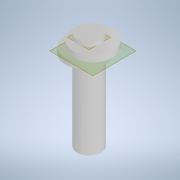
# Autodesk Inventor part: input_shaft
Saved by Autodesk Inventor 2022 (Build 260153000, 153)
## iProperties
Created: 2021-07-18
Part Number: input_shaft
Material: Generic
Document SubType Name: Modeling
Designer: Madhav
Density: 1 g/cm^3
Appearance: Default
Author: Madhav
Autodesk Inventor part; units mm, degrees
ref_plane "YZ Plane" through (0, 0, 0) normal (1, 0, 0) x (0, 1, 0)
ref_plane "XZ Plane" through (0, 0, 0) normal (0, 1, 0) x (-1, 0, 0)
ref_plane "XY Plane" through (0, 0, 0) normal (0, 0, 1) x (1, 0, 0)
sketch "Sketch1" plane through (0, 0, 0) normal (0, 1, 0) x (-1, 0, 0)
  point P0 (0, 0)
sketch "Sketch2" plane through (0, 0, 0) normal (0, 1, 0) x (-1, 0, 0)
  circle A0 centre (0, 0) radius 6
  dimension "d20" = 12
  constraints: 1 centre point, 1 coincident
  measures "d20" diameter of A0
extrude "Extrusion1" add sketch "Sketch2" along normal blind 50
ref_plane "Work Plane1" through (0, 48, 0) normal (0, 1, 0) x (1, 0, 0)
sketch "Sketch3" plane through (0, 48, 0) normal (0, 1, 0) x (1, 0, 0)
  line L0 (0, 0) -> (2, 0)
  circle A0 centre (2, 0) radius 10
  dimension "d4" = 2
  dimension "d5" = 20
  constraints: 2 end point, 1 centre point, 1 coincident, 1 horizontal
  measures "d4" distance of L0.start L0.end
  measures "d5" diameter of A0
extrude "Extrusion2" add sketch "Sketch3" against normal blind 3
ref_plane "Work Plane2" through (2, 43, 0) normal (0, -1, 0) x (1, 0, 0)
sketch "Sketch5" plane through (2, 43, 0) normal (0, -1, 0) x (1, 0, 0)
  line L0 (-2, 0) -> (-4, 0)
  circle A0 centre (-4, 0) radius 10
  dimension "d16" = 2
  dimension "d17" = 20
  constraints: 2 end point, 1 centre point, 1 coincident, 1 horizontal
  measures "d16" distance of L0.start L0.end
  measures "d17" diameter of A0
extrude "Extrusion4" add sketch "Sketch5" along normal blind 3
sketch "Sketch6" plane through (0, 0, 0) normal (0, -1, 0) x (1, 0, 0)
  circle A0 centre (0, 0) radius 3.5
  arc A1 (4.2426, 1.5) -> (4.2426, -1.5) centre (0, 0) ccw
  line L0 (5.4, 1.5) -> (4.2426, 1.5)
  line L1 (4.2426, -1.5) -> (5.4, -1.5)
  line L2 (5.4, -1.5) -> (5.4, 1.5)
  point P0 (0, 0)
  point P1 (0, 0)
  constraints: 6 end point, 2 centre point, 2 point on circle, 2 other
extrude "Extrusion5" cut sketch "Sketch6" against normal blind 4 contours A0 | L0 L2 L1 A1
fillet "Fillet1" radius 1 1 edges at (-4.5, 0, 0)
body "Solid1"
